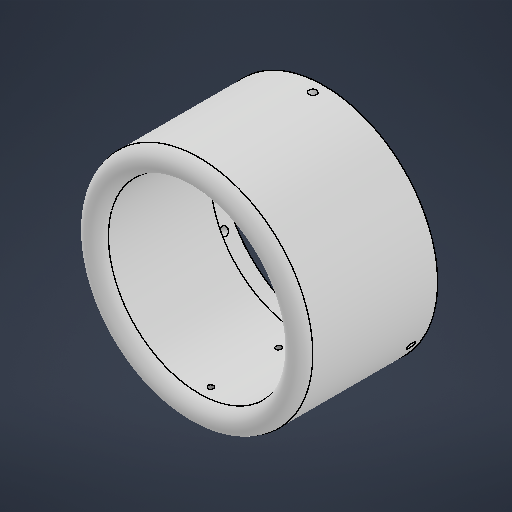
# Autodesk Inventor part: Nose
Saved by Autodesk Inventor 2026.1 (Build 301233000, 233)
## iProperties
Created: 2025-09-27
Part Number: Nose
Material: Generic
Document SubType Name: Modeling
Designer: 1char
Mass: 152.748 g
Surface Area: 389.283 cm^2
Volume: 152.748 cm^3
Density: 1 g/cm^3
Appearance: Default
Author: 1char
Autodesk Inventor part; units mm, degrees
ref_plane "YZ Plane" through (0, 0, 0) normal (1, 0, 0) x (0, 1, 0)
ref_plane "XZ Plane" through (0, 0, 0) normal (0, 1, 0) x (-1, 0, 0)
ref_plane "XY Plane" through (0, 0, 0) normal (0, 0, 1) x (1, 0, 0)
sketch "Sketch1" plane through (0, 0, 0) normal (0, 0, 1) x (1, 0, 0)
  circle A0 centre (0, 0) radius 40
  circle A1 centre (0, 0) radius 50
  dimension "d0" = 80
  dimension "d1" = 100
  constraints: 2 centre point, 2 coincident
  measures "d0" diameter of A0
  measures "d1" diameter of A1
extrude "Extrusion1" add sketch "Sketch1" along normal blind 50
sketch "Sketch2" plane through (0, 0, 0) normal (0, 0, -1) x (-1, 0, 0)
  circle A0 centre (0, 0) radius 45.1
  circle A1 centre (0, 0) radius 50 projected
  dimension "d5" = 90.2
  constraints: 1 centre point, 1 coincident
  measures "d5" diameter of A0
extrude "Extrusion2" add sketch "Sketch2" along normal blind 10
sketch "Sketch3" plane through (0, 0, 0) normal (0, 1, 0) x (-1, 0, 0)
  line L0 (-50, -10) -> (50, -10) construction
  point P0 (0, 0)
  point P1 (0, -5)
  dimension "d8" = 5
  constraints: 1 vertical alignment
  measures "d8" distance from line of L0 point (0, -5)
hole "Hole1" at (0, 0, -5) direction (0, 1, 0) diameter 3.4 end through all clearance for "Socket Head Cap Screw DIN EN ISO 4762" size "M3" standard "DIN"
pattern_circular "Circular Pattern1" count 3 over 360 about axis through (0, 0, -10) along (0, 0, 1) of "Hole1"
fillet "Fillet1" radius 5 2 edges at (-50, 0, 50) (-40, 0, 50)
sketch "Sketch4" plane through (0, 0, 0) normal (0, 1, 0) x (-1, 0, 0)
  point P0 (0, 0)
  point P1 (0, 40)
  point P2 (0, 10)
  dimension "d19" = 10
  dimension "d20" = 40
  constraints: 2 vertical alignment
  measures "d19" distance of point (0, 10) point (0, 0)
  measures "d20" distance of point (0, 0) point (0, 40)
hole "Hole2" at (0, 0, 40) at (0, 0, 10) direction (0, -1, 0) diameter 2.459 end through all thread size "M3x0.5" class "6H" standard "ANSI Metric M Profile"
body "Solid1"
